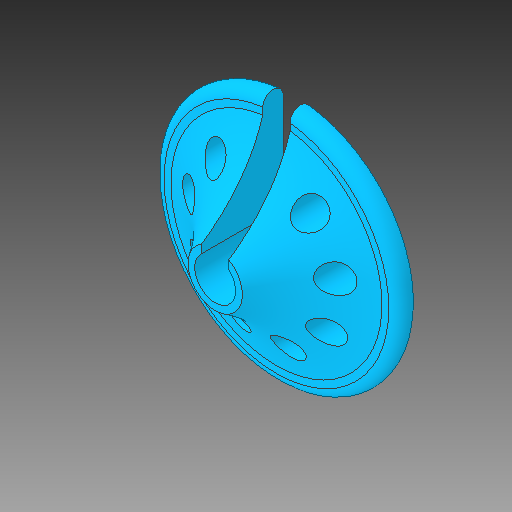
# Autodesk Inventor part: タミヤダンパー10
Saved by Autodesk Inventor 2019.2 (Build 232265000, 265)
## iProperties
Part Number: タミヤダンパー10
Material: 一般
Document SubType Name: Modeling
Designer: 雪村
Density: 1 g/cm^3
Appearance: 既定
Author: 雪村
Autodesk Inventor part; units mm, degrees
ref_plane "YZ Plane" through (0, 0, 0) normal (1, 0, 0) x (0, 1, 0)
ref_plane "XZ Plane" through (0, 0, 0) normal (0, 1, 0) x (-1, 0, 0)
ref_plane "XY Plane" through (0, 0, 0) normal (0, 0, 1) x (1, 0, 0)
sketch "スケッチ1" plane through (0, 0, 0) normal (0, 0, 1) x (1, 0, 0)
  circle A0 centre (0, 0) radius 9
  dimension "d0" = 18
  constraints: 1 centre point, 1 coincident
  measures "d0" diameter of A0
extrude "押し出し1" add sketch "スケッチ1" along normal blind 1.5
fillet "フィレット1" radius 0.75 2 edges at (-9, 0, 1.5) (-9, 0, 0)
sketch "スケッチ3" plane through (0, 0, 0) normal (0, 1, 0) x (-1, 0, 0)
  line L0 (-8.25, 1.5) -> (8.25, 1.5) projected
  line L1 (8.25, 0) -> (-8.25, 0) projected
  line L2 (0, 0) -> (0, 6)
  line L3 (-8.25, 1.5) -> (8.25, 1.5) projected
  arc A0 (2, 6) -> (7.75, 1.5) centre (10.6127, 11.0815) ccw
  arc A1 (-7.75, 1.5) -> (-2, 6) centre (-10.6127, 11.0815) ccw
  line L4 (2, 6) -> (0, 6)
  dimension "d5" = 6
  dimension "d6" = 2
  dimension "d7" = 2
  dimension "d8" = 10
  dimension "d9" = 10
  dimension "d10" = 7.75
  dimension "d11" = 7.75
  constraints: 4 end point, 4 point on circle, 2 centre point, 2 horizontal alignment, 2 point on line, 1 vertical
  measures "d5" distance of L2.start L2.end
  measures "d6" distance of L2.end L4.start
  measures "d7" distance from line of A1.end L2
  measures "d8" radius of A0
  measures "d9" radius of A1
  measures "d10" distance from line of L2 A0.end
  measures "d11" distance from line of L2 A1.start
revolve "回転1" add sketch "スケッチ3" angle 360 about axis through (0, 0, 0) along (0, 0, 1) fills toward (0.05, 3) open curves L2 L4 A0
sketch "スケッチ4" plane through (0, 0, 0) normal (0, 0, -1) x (-1, 0, 0)
  line L0 (1.875, -5.1515) -> (-1.875, -5.1515) construction
  line L1 (-1.875, -5.1515) -> (-4.7477, -2.7411) construction
  line L2 (-4.7477, -2.7411) -> (-5.3988, 0.952) construction
  line L3 (-5.3988, 0.952) -> (-3.5238, 4.1996) construction
  line L4 (-3.5238, 4.1996) -> (0, 5.4821) construction
  line L5 (0, 5.4821) -> (3.5238, 4.1996) construction
  line L6 (3.5238, 4.1996) -> (5.3988, 0.952) construction
  line L7 (5.3988, 0.952) -> (4.7477, -2.7411) construction
  line L8 (4.7477, -2.7411) -> (1.875, -5.1515) construction
  circle A0 centre (3.5238, 4.1996) radius 1
  circle A1 centre (0, 0) radius 1.5
  circle A2 centre (5.3988, 0.952) radius 1
  circle A3 centre (4.7477, -2.7411) radius 1
  circle A4 centre (1.875, -5.1515) radius 1
  circle A5 centre (-1.875, -5.1515) radius 1
  circle A6 centre (-4.7477, -2.7411) radius 1
  circle A7 centre (-5.3988, 0.952) radius 1
  circle A8 centre (-3.5238, 4.1996) radius 1
  dimension "d14" = 3.75
  dimension "d15" = 2
  dimension "d16" = 3
  dimension "d17" = 2
  dimension "d18" = 2
  dimension "d19" = 2
  dimension "d20" = 2
  dimension "d21" = 2
  dimension "d22" = 2
  dimension "d23" = 2
  constraints: 18 end point, 10 coincident, 9 centre point, 1 horizontal, 19 other
  measures "d14" distance of L0.start L0.end
  measures "d15" diameter of A0
  measures "d16" diameter of A1
  measures "d17" diameter of A2
  measures "d18" diameter of A3
  measures "d19" diameter of A4
  measures "d20" diameter of A5
  measures "d21" diameter of A6
  measures "d22" diameter of A7
  measures "d23" diameter of A8
extrude "押し出し2" cut sketch "スケッチ4" against normal through all
sketch "スケッチ5" plane through (0, 0, 0) normal (0, 0, -1) x (-1, 0, 0)
  arc A0 (-1, 2.2913) -> (1, 2.2913) centre (0, 0) ccw construction
  line L0 (1, 1.118) -> (1, 10.0764)
  line L1 (-1, 1.118) -> (-1, 10.0764)
  line L2 (1, 10.0764) -> (-1, 10.0764)
  line L3 (0, 0) -> (0, 10.0764) construction
  circle A1 centre (0, 0) radius 1.5 projected
  dimension "d26" = 5
  dimension "d27" = 2
  constraints: 8 end point, 4 point on circle, 3 vertical, 2 point on line, 1 centre point, 1 coincident, 1 horizontal, 1 midpoint
  measures "d26" diameter of A0
  measures "d27" distance between parallel lines of L1 L0
extrude "押し出し4" cut sketch "スケッチ5" against normal through all contours A1 L1 L2 L0
equation "\"d9\" = d8"
equation "\"d11\" = d10"
